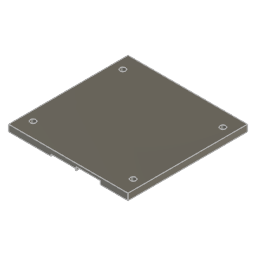
sample_stage (Autodesk Fusion 360 design; units mm, degrees)
part number: 2026-04-23-15-36-49-562
Autodesk Fusion 360 part; units mm, degrees
note: some values were not read from the file. Chosen so that the rebuilt part matches the saved one: which face or edge a step refers to. Set by a fixed rule: which sketch regions a step uses.
sketch "Sketch1" plane through (0, 0, 0) normal (0, 0, 1) x (1, 0, 0)
  line L0 (-27.3, 27.3) -> (27.3, 27.3)
  line L1 (27.3, 27.3) -> (27.3, -27.3)
  line L2 (27.3, -27.3) -> (-27.3, -27.3)
  line L3 (-27.3, -27.3) -> (-27.3, 27.3)
  line L4 (-27.3, 27.3) -> (27.3, -27.3) construction
  line L5 (27.3, 27.3) -> (-27.3, -27.3) construction
  circle A0 centre (-22.85, 20.5) radius 1.25
  circle A1 centre (-22.85, -20.5) radius 1.25
  circle A2 centre (22.85, 20.5) radius 1.25
  circle A3 centre (22.85, -20.5) radius 1.25
  circle A4 centre (-5, 20) radius 1.25
  circle A5 centre (5, 20) radius 1.25
  circle A6 centre (-17.35, 20.5) radius 1.25
  circle A7 centre (-17.35, -20.5) radius 1.25
  circle A8 centre (17.35, -20.5) radius 1.25
  circle A9 centre (17.35, 20.5) radius 1.25
  dimension "d1" = 54.6
  dimension "d2" = 2.5
  dimension "d3" = 41
  dimension "d9" = 2.5
  dimension "d10" = 20
  dimension "d11" = 5
  dimension "d12" = 5
  dimension "d16" = 5.5
  dimension "d17" = 5.5
  dimension "d34" = 45.7
  dimension "d42" = 22.85
  dimension "d43" = 20.5
  constraint horizontal L0
  constraint perpendicular L0 L1
  constraint parallel L0 L2
  constraint parallel L1 L3
  constraint coincident L4 origin
  constraint coincident L5 origin
  constraint equal L0 L3
  constraint vertical A0.centre A1.centre
  constraint horizontal A1.centre A3.centre
  constraint vertical A2.centre A3.centre
  constraint horizontal A0.centre A2.centre
  constraint equal A0 A1
  constraint equal A1 A3
  constraint equal A2 A3
  constraint equal A4 A5
  constraint horizontal A4.centre A5.centre
  constraint equal A6 A9
  constraint equal A2 A9
  constraint equal A2 A8
  constraint equal A7 A8
  constraint horizontal A0.centre A6.centre
  constraint vertical A6.centre A7.centre
  constraint horizontal A1.centre A7.centre
  constraint horizontal A7.centre A8.centre
  constraint vertical A8.centre A9.centre
  constraint horizontal A2.centre A9.centre
  measures "d1" distance of L0.start L0.end
  measures "d2" diameter of A0
  measures "d3" distance of A0.centre A1.centre
  measures "d9" diameter of A4
  measures "d10" vertical distance of origin A4.centre
  measures "d11" horizontal distance of origin A4.centre
  measures "d12" horizontal distance of origin A5.centre
  measures "d16" distance of A0.centre A6.centre
  measures "d17" distance of A2.centre A9.centre
  measures "d34" distance of A0.centre A2.centre
  measures "d42" horizontal distance of origin A0.centre
  measures "d43" vertical distance of origin A0.centre
extrude "Extrude1" add sketch "Sketch1" along normal blind 3 contours L0 L1 L2 L3 | A4 | A5 | A6 | A7 | A8 | A9
sketch "Sketch9" plane through (0, -27.3, 0) normal (0, -1, 0) x (1, 0, 0)
  line L0 (-27.3, 0) -> (27.3, 0)
  line L1 (27.3, 0) -> (27.3, 3)
  line L2 (27.3, 3) -> (-27.3, 3)
  line L3 (-27.3, 3) -> (-27.3, 0)
  line L4 (-3.1, 0) -> (-3.25, 0.3)
  line L5 (-3.25, 0.3) -> (3.25, 0.3)
  line L6 (3.25, 0.3) -> (3.1, 0)
  dimension "d44" = 0.15
  dimension "d45" = 0.3
  dimension "d46" = 6.5
  dimension "d56" = 3.25
  constraint coincident L0 L4.start
  constraint parallel L0 L5
  constraint coincident L0 L6.end
  constraint equal L4 L6
  measures "d44" horizontal distance of L5.end L6.end
  measures "d45" vertical distance of L5.end L6.end
  measures "d46" distance of L4.end L5.end
  measures "d56" horizontal distance of origin L4.end
extrude "Extrude7" cut sketch "Sketch9" against normal blind 55 contours L0 L4 L5 L6
sketch "Sketch10" plane through (0, 0, 0) normal (0, 0, -1) x (1, 0, 0)
  line L0 (-3.1, -27.3) -> (-3.1, 27.3)
  line L1 (-3.1, 27.3) -> (-27.3, 27.3)
  line L2 (-27.3, 27.3) -> (-27.3, -27.3)
  line L3 (-27.3, -27.3) -> (-3.1, -27.3)
  line L4 (27.3, -27.3) -> (27.3, 27.3)
  line L5 (27.3, 27.3) -> (3.1, 27.3)
  line L6 (3.1, 27.3) -> (3.1, -27.3)
  circle A0 centre (-22.85, 20.5) radius 1.25
  circle A1 centre (-22.85, -20.5) radius 1.25
  circle A2 centre (22.85, -20.5) radius 1.25
  circle A3 centre (22.85, 20.5) radius 1.25
  line L7 (14.6, -27.3) -> (3.6, -27.3)
  line L8 (3.6, -27.3) -> (3.6, 27.7)
  line L9 (3.6, 27.7) -> (14.6, 27.7)
  line L10 (14.6, 27.7) -> (14.6, -27.3)
  line L11 (3.1, -27.3) -> (27.3, -27.3)
  dimension "d50" = 11
  dimension "d51" = 55
  dimension "d53" = 0.5
  constraint horizontal L7
  constraint vertical L8
  constraint horizontal L9
  constraint vertical L10
  constraint coincident L3 L7.start
  measures "d50" distance of L8.end L9.end
  measures "d51" distance of L7.start L9.end
  measures "d53" distance of L6 L8
extrude "Extrude8" cut sketch "Sketch10" against normal blind 1.6 contours L5 L7 L8 L10 L11 | L5 L8 L9 L10
sketch "Sketch11" plane through (0, 0, 0) normal (0, 0, -1) x (1, 0, 0)
  line L0 (27.3, 27.3) -> (14.6, 27.3)
  line L1 (-3.1, -27.3) -> (-3.1, 27.3)
  line L2 (-3.1, 27.3) -> (-27.3, 27.3)
  line L3 (-27.3, 27.3) -> (-27.3, -27.3)
  line L4 (-27.3, -27.3) -> (-3.1, -27.3)
  circle A0 centre (-22.85, 20.5) radius 1.25
  circle A1 centre (-22.85, -20.5) radius 1.25
  line L5 (3.1, -27.3) -> (-7.9, -27.3)
  line L6 (-7.9, -27.3) -> (-7.9, 27.3)
  line L7 (-7.9, 27.3) -> (3.1, 27.3)
  line L8 (3.1, 27.3) -> (3.1, -27.3)
  line L9 (14.6, 27.3) -> (14.6, -27.3)
  line L10 (14.6, -27.3) -> (27.3, -27.3)
  line L11 (27.3, -27.3) -> (27.3, 27.3)
  circle A2 centre (22.85, -20.5) radius 1.25
  circle A3 centre (22.85, 20.5) radius 1.25
  line L12 (3.25, -27.3) -> (-3.25, -27.3)
  dimension "d57" = 4.8
  constraint horizontal L5
  constraint vertical L6
  constraint horizontal L7
  constraint vertical L8
  constraint coincident L2 L6.end
  constraint collinear L5 L12
  measures "d57" distance of L1 L6
extrude "Extrude9" cut sketch "Sketch11" against normal blind 0.8 contours L1 L2 L4 L5 L6 L7 L12 | L1 L5 L7 L8 L12
sketch "Sketch5" plane through (0, 0, 0) normal (0, 0, -1) x (1, 0, 0)
  line L0 (25, 25) -> (-25, 25)
  line L1 (-25, 25) -> (-25, -25)
  line L2 (-25, -25) -> (25, -25)
  line L3 (25, -25) -> (25, 25)
  circle A0 centre (-15.15, -20.5) radius 1.25
  circle A1 centre (20.65, 20.5) radius 1.25
  circle A2 centre (-20.65, -20.5) radius 1.25
  circle A3 centre (-15.15, 20.5) radius 1.25
  circle A4 centre (20.65, -20.5) radius 1.25
  circle A5 centre (15.15, -20.5) radius 1.25
  circle A6 centre (15.15, 20.5) radius 1.25
  circle A7 centre (-20.65, 20.5) radius 1.25
  line L4 (25, -25) -> (-25, -25)
  line L5 (-25, -25) -> (-25, 25)
  line L6 (-25, 25) -> (25, 25)
  line L7 (25, 25) -> (25, -25)
  constraint horizontal L4
  constraint vertical L5
  constraint horizontal L6
  constraint vertical L7
  constraint coincident L0.end L1.start
  constraint coincident L2.end L3.start
sketch "Sketch6" plane through (0, 0, 3) normal (0, 0, 1) x (-1, 0, 0)
  line L0 (27.5, 27.5) -> (-27.5, 27.5)
  line L1 (-27.5, 27.5) -> (-27.5, -27.5)
  line L2 (-27.5, -27.5) -> (27.5, -27.5)
  line L3 (27.5, -27.5) -> (27.5, 27.5)
  circle A0 centre (23.15, 20.5) radius 1.25
  circle A1 centre (23.15, -20.5) radius 1.25
  line L4 (-27.5, -12.8) -> (27.5, -12.8)
  line L5 (27.5, -12.8) -> (27.5, 12.8)
  line L6 (27.5, 12.8) -> (-27.5, 12.8)
  line L7 (-27.5, 12.8) -> (-27.5, -12.8)
  line L8 (-27.5, -12.8) -> (27.5, 12.8) construction
  line L9 (27.5, -12.8) -> (-27.5, 12.8) construction
  circle A2 centre (-23.15, 20.5) radius 1.25
  circle A3 centre (-23.15, -20.5) radius 1.25
  dimension "d23" = 25.6
  constraint horizontal L4
  constraint perpendicular L4 L5
  constraint parallel L4 L6
  constraint parallel L5 L7
  constraint coincident L8 origin
  constraint coincident L9 origin
  constraint coincident L1 L4.start
  measures "d23" distance of L4.start L6.end
extrude "Extrude4" [suppressed]
sketch "Sketch7" plane through (0, 0, 0) normal (0, 0, -1) x (1, 0, 0)
  line L0 (27.5, 27.5) -> (-27.5, 27.5)
  line L1 (-27.5, 27.5) -> (-27.5, -27.5)
  line L2 (-27.5, -27.5) -> (27.5, -27.5)
  line L3 (27.5, -27.5) -> (27.5, 27.5)
  circle A0 centre (-23.15, 20.5) radius 1.25
  circle A1 centre (-23.15, -20.5) radius 1.25
  circle A2 centre (17.5, -20.4) radius 1.5
  circle A3 centre (-17.5, -20.4) radius 1.5
  circle A4 centre (17.5, 20.4) radius 1.5
  circle A5 centre (-17.5, 20.4) radius 1.5
  circle A6 centre (23.15, 20.5) radius 1.25
  circle A7 centre (23.15, -20.5) radius 1.25
  dimension "d26" = 35
  dimension "d27" = 40.8
  dimension "d28" = 3
  dimension "d29" = 20.4
  dimension "d30" = 17.5
  constraint equal A4 A5
  constraint equal A2 A4
  constraint equal A2 A3
  constraint vertical A2.centre A4.centre
  constraint horizontal A4.centre A5.centre
  constraint vertical A3.centre A5.centre
  constraint horizontal A2.centre A3.centre
  measures "d26" distance of A2.centre A3.centre
  measures "d27" distance of A2.centre A4.centre
  measures "d28" diameter of A4
  measures "d29" vertical distance of origin A4.centre
  measures "d30" horizontal distance of origin A2.centre
extrude "Extrude5" [suppressed]
sketch "Sketch8" plane through (0, 0, 6) normal (0, 0, 1) x (-1, 0, 0)
  line L0 (-27.5, 12.8) -> (-27.5, -12.8)
  line L1 (-27.5, -12.8) -> (27.5, -12.8)
  line L2 (27.5, -12.8) -> (27.5, 12.8)
  line L3 (27.5, 12.8) -> (-27.5, 12.8)
  circle A0 centre (25, -5) radius 1.5
  circle A1 centre (25, 5) radius 1.5
  circle A2 centre (9.3, 5) radius 1.5
  circle A3 centre (9.3, -5) radius 1.5
  dimension "d35" = 15.7
  dimension "d36" = 10
  dimension "d37" = 3
  dimension "d38" = 5
  dimension "d39" = 2.5
  constraint vertical A0.centre A1.centre
  constraint horizontal A1.centre A2.centre
  constraint vertical A2.centre A3.centre
  constraint horizontal A0.centre A3.centre
  constraint equal A2 A3
  constraint equal A1 A2
  constraint equal A0 A1
  measures "d35" horizontal distance of A0.centre A3.centre
  measures "d36" vertical distance of A0.centre A1.centre
  measures "d37" diameter of A0
  measures "d38" vertical distance of origin A3.centre
  measures "d39" distance of L2 A0.centre
extrude "Extrude6" [suppressed]
equation "d2 = d9"
equation "d5 = 20 mm - 2.1 mm"
equation "d12 = d11"
equation "d17 = d16"
equation "d29 = d27 / 2"
equation "d30 = d26 / 2"
equation "d38 = d36 / 2"
equation "d42 = d34 / 2"
equation "d43 = d3 / 2"
equation "d56 = d46 / 2"
equation "d57 = 11 mm - 6.2 mm"
